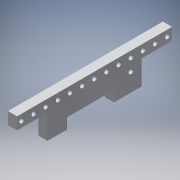
# Autodesk Inventor part: SpanRearAndMiddleSupport
Saved by Autodesk Inventor 2016 SP1 (Build 200210100, 210)
## iProperties
Created: 2016-02-14
Part Number: SpanRearAndMiddleSupport
Material: Aluminum 6061
Document SubType Name: Modeling
Designer: steele
Density: 2.7 g/cm^3
Appearance: Aluminum - Flat
Mass: 628.65 g
Surface Area: 453.434 cm^2
Volume: 232.833 cm^3
Author: steele
Autodesk Inventor part; units mm, degrees
ref_plane "YZ Plane" through (0, 0, 0) normal (1, 0, 0) x (0, 1, 0)
ref_plane "XZ Plane" through (0, 0, 0) normal (0, 1, 0) x (-1, 0, 0)
ref_plane "XY Plane" through (0, 0, 0) normal (0, 0, 1) x (1, 0, 0)
sketch "Sketch2" plane through (0, 0, 0) normal (1, 0, 0) x (0, 1, 0)
  line L0 (0, 0) -> (0, 95.25)
  line L1 (0, 95.25) -> (50.8, 95.25)
  line L2 (50.8, 95.25) -> (50.8, 158.75)
  line L3 (50.8, 158.75) -> (76.2, 158.75)
  line L4 (76.2, 158.75) -> (76.2, 15.0657)
  line L5 (76.2, 15.0657) -> (76.2, 0)
  line L6 (76.2, 0) -> (0, 0) construction
  line L7 (0, 0) -> (0, -95.25)
  line L8 (0, -95.25) -> (50.8, -95.25)
  line L9 (50.8, -95.25) -> (50.8, -158.75)
  line L10 (50.8, -158.75) -> (76.2, -158.75)
  line L11 (76.2, -158.75) -> (76.2, -15.0657)
  line L12 (76.2, -15.0657) -> (76.2, 0)
  dimension "d5" = 50.8
  dimension "d6" = 25.4
  dimension "d8" = 63.5
  dimension "d9" = 95.25
  constraints: 26 end point, 5 symmetric about line, 3 perpendicular, 3 vertical, 1 horizontal
  measures "d5" distance of L0.end L1.end
  measures "d6" distance of L2.end L3.end
  measures "d8" distance of L1.end L2.end
  measures "d9" distance of L0.start L0.end
extrude "Extrusion1" add sketch "Sketch2" along normal mid plane 19.05
sketch "Sketch3" plane through (9.525, 50.8, -95.25) normal (0, 0, -1) x (-1, 0, 0)
  line L0 (19.05, 0) -> (19.05, 25.4) projected
  line L1 (0, -50.8) -> (19.05, -50.8)
  line L2 (19.05, -50.8) -> (19.05, 0)
  line L3 (19.05, 0) -> (0, 0)
  line L4 (0, 0) -> (0, -50.8)
  point P0 (9.525, -50.8)
  constraints: 8 end point, 2 parallel, 1 horizontal, 1 perpendicular
extrude "Extrusion2" add sketch "Sketch3" along normal blind 6.35
sketch "Sketch4" plane through (9.525, 76.2, -158.75) normal (0, 0, -1) x (-1, 0, 0)
  line L0 (0, 0) -> (0, -25.4) projected
  line L1 (19.05, -25.4) -> (19.05, 0) projected
  line L2 (0, 0) -> (19.05, 0)
  line L3 (19.05, 0) -> (19.05, -25.4)
  line L4 (19.05, -25.4) -> (0, -25.4)
  line L5 (0, -25.4) -> (0, 0)
  point P0 (9.525, -76.2)
  constraints: 8 end point, 2 parallel, 1 horizontal, 1 perpendicular
extrude "Extrusion3" add sketch "Sketch4" along normal blind 6.35
sketch "Sketch6" plane through (9.525, 0, 0) normal (1, 0, 0) x (0, 0, -1)
  line L0 (-95.25, 50.8) -> (-95.25, 0) construction
  line L1 (-95.25, 38.1) -> (101.6, 38.1) construction
  line L2 (101.6, 50.8) -> (101.6, 0) construction
  line L3 (-158.75, 76.2) -> (165.1, 76.2) construction
  circle A0 centre (79.375, 38.1) radius 4.7625
  line L4 (165.1, 76.2) -> (165.1, 50.8) projected
  point P0 (0, 0)
  dimension "d28" = 38.1
  dimension "d29" = 85.725
  dimension "d30" = 9.525
  constraints: 3 point on line, 2 end point, 1 centre point, 1 horizontal
  measures "d28" distance between parallel lines of L1 L3
  measures "d29" distance from line of A0.centre L4
  measures "d30" diameter of A0
extrude "Extrusion5" cut sketch "Sketch6" against normal through all
sketch "Sketch7" plane through (9.525, 0, 0) normal (1, 0, 0) x (0, 0, -1)
  circle A0 centre (79.375, 38.1) radius 4.7625 projected
  line L0 (-95.25, 0) -> (101.6, 0) projected
  line L1 (-95.25, 0) -> (-95.25, 50.8) projected
  line L2 (-95.25, 50.8) -> (-158.75, 50.8) projected
  line L3 (-158.75, 50.8) -> (-158.75, 76.2) projected
  line L4 (-158.75, 76.2) -> (165.1, 76.2) projected
  line L5 (165.1, 50.8) -> (165.1, 76.2) projected
  line L6 (101.6, 50.8) -> (165.1, 50.8) projected
  line L7 (101.6, 0) -> (101.6, 50.8) projected
  line L8 (-95.25, 0) -> (101.6, 0) projected
  line L9 (-54.5452, 0) -> (43.8798, 0)
  line L10 (43.8798, 0) -> (43.8798, 22.225)
  line L11 (43.8798, 22.225) -> (-54.5452, 22.225)
  line L12 (-54.5452, 22.225) -> (-54.5452, 0)
  point P0 (0, 0)
  dimension "d33" = 98.425
  dimension "d34" = 22.225
  constraints: 8 end point, 2 parallel, 1 horizontal, 1 perpendicular, 1 point on line
  measures "d33" distance of L10.end L11.end
  measures "d34" distance of L11.end L9.start
extrude "Extrusion6" cut sketch "Sketch7" against normal through all contours L12 L11 L10 L0
body "Solid1"
